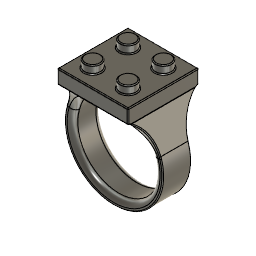
Ring Head (Autodesk Fusion 360 design; units mm, degrees)
Autodesk Fusion 360 part; units mm, degrees
note: some values were not read from the file. Set by a fixed rule: which face or edge a step refers to.
sketch "Sketch5" plane through (0, 0, 0) normal (0, 1, 0) x (1, 0, 0) in component "Component"
  circle A0 centre (0, 0) radius 9.3
  line L0 (-10.4953, -3.6138) -> (-8, -10.8606)
  line L1 (-8, -10.8606) -> (8, -10.8606)
  line L2 (8, -10.8606) -> (10.4953, -3.6138)
  line L3 (0, -1.75) -> (0, -22.5)
  arc A1 (10.4953, -3.6138) -> (-10.4953, -3.6138) centre (0, 0) ccw
  dimension "d24" = 18.6
  dimension "d26" = 19
  dimension "d27" = 16
  constraint coincident A0.centre A1.centre
  constraint horizontal L1
  constraint tangent L0 A1
  constraint tangent L2 A1
  constraint symmetric L0 L2 L3
  measures "d24" diameter of A0
  measures "d26" angle of L0 L3
  measures "d27" distance of L0.end L1.end
extrude "Extrude3" add sketch "Sketch5" along normal mid plane 16 in component "Component"
ref_plane "WorkPlane1" through (0, 0, 14.2) normal (0, 0, 1) x (1, 0, 0) in component "Component"
extrude "Extrude4" add 1 faces at (-2.6667, -2.6667, 10.8606) along direction (0, 0, 1) up to surface (3.3394 mm away) in component "Component"
sketch "Sketch6" plane through (0, 0, 0) normal (1, 0, 0) x (0, 1, 0) in component "Component"
  line L0 (8, 11.05) -> (8, -11.1)
  line L1 (8, -11.1) -> (3.25, -11.1)
  line L2 (3.25, -11.1) -> (3.25, 3.1167)
  arc A0 (8, 11.05) -> (3.25, 3.1167) centre (12.25, 3.1167) ccw
  line L3 (0, 2.5) -> (0, 20)
  line L4 (-8, 11.05) -> (-8, -11.1)
  line L5 (-3.25, -11.1) -> (-3.25, 3.1167)
  arc A1 (-3.25, 3.1167) -> (-8, 11.05) centre (-12.25, 3.1167) ccw
  line L6 (-8, -11.1) -> (-3.25, -11.1)
  dimension "d33" = 3.25
  dimension "d34" = 8
  dimension "d35" = 11.1
  dimension "d36" = 22.15
  dimension "d37" = 9
  constraint horizontal L1
  constraint perpendicular L1 L2
  constraint vertical L0
  constraint tangent L2 A0
  constraint symmetric L0.start L3 L4.start
  constraint symmetric L0.end L3 L4.end
  constraint symmetric L1.end L3 L5.start
  constraint symmetric L2.end L3 L5.end
  constraint symmetric A0 L3 A1
  measures "d33" distance of origin L2
  measures "d34" distance of origin L0
  measures "d35" distance of origin L1
  measures "d36" distance of L0.start L0.end
  measures "d37" radius of A0
extrude "Extrude5" cut sketch "Sketch6" along normal through all and the other way through all in component "Component"
sketch "Sketch7" plane through (0, 0, 14.2) normal (0, 0, 1) x (-1, 0, 0) in component "Component"
  line L0 (8, 8) -> (-8, 8)
  line L1 (-8, 8) -> (-8, -8)
  line L2 (-8, -8) -> (8, -8)
  line L3 (8, -8) -> (8, 8)
  circle A0 centre (-4, 4) radius 1.8259
  dimension "d39" = 4
  dimension "d40" = 4
  measures "d39" horizontal distance of origin A0.centre
  measures "d40" vertical distance of origin A0.centre
extrude "Extrude6" add sketch "Sketch7" along normal blind 1.8 contours A0 in component "Component"
pattern_linear "R-Pattern1" count 2 spacing 8 along (-1, 0, 0) count 2 spacing 8 along (0, 1, 0) of "Extrude6" in component "Component"
fillet "Fillet1" radius 1.2 2 edges at (0, -3.25, -9.3) (0, -5.7104, 9.3) in component "Component"
fillet "Fillet2" radius 1.2 2 edges at (0, 5.7104, 9.3) (0, 3.25, -9.3) in component "Component"
fillet "Fillet3" radius 0.2 10 edges at (9.0581, -4.5571, 7.7877) (10.5773, -3.2535, 3.366) (0, -3.25, -11.1) (-10.5773, -3.2535, 3.366) (-9.0581, -4.5571, 7.7877) (-9.0581, 4.5571, 7.7877) (-10.5773, 3.2535, 3.366) (0, 3.25, -11.1) (10.5773, 3.2535, 3.366) (9.0581, 4.5571, 7.7877) 8 faces at (8, -2.5546, 13.0869) (-2.6667, -8, 12.1) (-2.6667, 8, 12.1) (-8, -2.5546, 13.0869) (2.1831, -3.8182, 14.8) (2.1831, 4.1818, 14.8) (-5.8169, -3.8182, 14.8) (-5.8169, 4.1818, 14.8) in component "Component"
component "Component" placed x (1, 0, 0) y (0, 1, 0) z (0, 0, 1) at (0, 0, 0)
equation "d33 = ( 6.5 / 2 ) * 1 mm"
